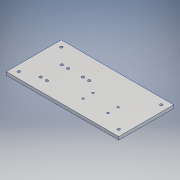
# Autodesk Inventor part: Plaque support
Saved by Autodesk Inventor 2017 (Build 210142000, 142)
## iProperties
Part Number: Plaque support
Material: Aluminium 6061
Document SubType Name: Modeling
Designer: Adrien MARY
Density: 2.7 g/cm^3
Appearance: Aluminium - Plat
Mass: 211.535 g
Surface Area: 348.794 cm^2
Volume: 78.3464 cm^3
Stock Number: 1410-02-01
Project: 1410 LaserShow
Author: Adrien MARY
Autodesk Inventor part; units mm, degrees
ref_plane "YZ Plane" through (0, 0, 0) normal (1, 0, 0) x (0, 1, 0)
ref_plane "XZ Plane" through (0, 0, 0) normal (0, 1, 0) x (-1, 0, 0)
ref_plane "XY Plane" through (0, 0, 0) normal (0, 0, 1) x (1, 0, 0)
sketch "Esquisse1" plane through (0, 0, 0) normal (0, 0, 1) x (1, 0, 0)
  line L0 (-90, -44) -> (90, -44)
  line L1 (90, -44) -> (90, 44)
  line L2 (90, 44) -> (-90, 44)
  line L3 (-90, 44) -> (-90, -44)
  line L4 (-90, -44) -> (90, 44) construction
  line L5 (90, -44) -> (-90, 44) construction
  point P0 (0, 0)
  dimension "d0" = 180
  dimension "d1" = 88
  constraints: 12 end point, 2 midpoint, 2 parallel, 1 horizontal, 1 perpendicular
  measures "d0" distance of L2.end L1.end
  measures "d1" distance of L1.end L0.end
extrude "Extrusion1" add sketch "Esquisse1" along normal mid plane 5
sketch "Esquisse2" plane through (0, 0, 2.5) normal (0, 0, 1) x (1, 0, 0)
  line L0 (-90, 44) -> (-90, -44) projected
  line L1 (90, -44) -> (-90, -44) projected
  point P0 (0, 0)
  point P1 (-45, -24)
  point P2 (-45, 9.85)
  point P3 (-11.15, 9.85)
  dimension "d4" = 33.85
  dimension "d5" = 45
  dimension "d6" = 33.85
  dimension "d7" = 20
  constraints: 1 horizontal alignment, 1 vertical alignment
  measures "d4" distance of point (-45, 9.85) point (-45, -24)
  measures "d5" distance from line of L0 point (-45, -24)
  measures "d6" distance of point (-45, 9.85) point (-11.15, 9.85)
  measures "d7" distance from line of L1 point (-45, -24)
hole "Perçage_moteur" at (-45, -24, 2.5) at (-45, 9.85, 2.5) at (-11.15, 9.85, 2.5) direction (0, 0, -1) diameter 4.2 end through all
sketch "Esquisse3" plane through (0, 0, 2.5) normal (0, 0, 1) x (1, 0, 0)
  line L0 (-60.0266, -12) -> (31.1582, -12) construction
  circle A0 centre (-45, -24) radius 2.1 construction
  circle A1 centre (-11.15, 9.85) radius 2.1 construction
  line L1 (-90, 44) -> (-90, -44) projected
  point P0 (0, 0)
  point P1 (8.85, -20)
  point P2 (8.85, -4)
  point P3 (48.85, -4)
  point P4 (48.85, -20)
  dimension "d15" = 40
  dimension "d16" = 16
  dimension "d17" = 12
  dimension "d18" = 8
  dimension "d19" = 20
  dimension "d38" = 98.85
  constraints: 2 end point, 2 horizontal alignment, 2 vertical alignment, 1 horizontal
  measures "d15" distance of point (48.85, -4) point (8.85, -4)
  measures "d16" distance of point (48.85, -20) point (48.85, -4)
  measures "d17" distance from line of L0 A0.centre
  measures "d18" distance from line of L0 point (8.85, -20)
  measures "d19" horizontal distance of A1.centre point (8.85, -4)
  measures "d38" distance from line of L1 point (8.85, -4)
hole "Perçage_laser" at (8.85, -20, 2.5) at (8.85, -4, 2.5) at (48.85, -4, 2.5) at (48.85, -20, 2.5) direction (0, 0, -1) diameter 3.2 depth 9.525 tip angle 118
sketch "Esquisse4" plane through (0, 0, 2.5) normal (0, 0, 1) x (1, 0, 0)
  line L0 (90, -44) -> (90, 44) projected
  line L1 (-90, 44) -> (90, 44) projected
  line L2 (90, -44) -> (-90, -44) projected
  line L3 (-90, 44) -> (-90, -44) projected
  point P0 (0, 0)
  point P1 (-80, -34)
  point P2 (-80, 34)
  point P3 (80, 34)
  point P4 (80, -34)
  dimension "d27" = 10
  dimension "d28" = 10
  dimension "d29" = 10
  dimension "d30" = 10
  constraints: 2 horizontal alignment, 2 vertical alignment
  measures "d27" distance from line of L0 point (80, 34)
  measures "d28" distance from line of L1 point (80, 34)
  measures "d29" distance from line of L2 point (80, -34)
  measures "d30" distance from line of L3 point (-80, -34)
hole "Perçage_coins" at (-80, -34, 2.5) at (-80, 34, 2.5) at (80, 34, 2.5) at (80, -34, 2.5) direction (0, 0, -1) diameter 4.2 depth 9.525 tip angle 118
sketch "Esquisse5" plane through (0, 0, 2.5) normal (0, 0, 1) x (1, 0, 0)
  circle A0 centre (-45, 9.85) radius 2.1 projected
  circle A1 centre (-11.15, 9.85) radius 2.1 projected
  circle A2 centre (-45, -24) radius 2.1 projected
  point P0 (0, 0)
  point P1 (-55, -24)
  point P2 (-55, 9.85)
  point P3 (-21.15, 9.85)
  dimension "d39" = 10
  dimension "d40" = 10
  dimension "d41" = 10
  constraints: 3 horizontal alignment
  measures "d39" distance of A0.centre point (-55, 9.85)
  measures "d40" distance of A1.centre point (-21.15, 9.85)
  measures "d41" distance of A2.centre point (-55, -24)
hole "Perçage4" at (-55, -24, 2.5) at (-55, 9.85, 2.5) at (-21.15, 9.85, 2.5) direction (0, 0, -1) diameter 4.2 depth 8 tip angle 118
equation "\"d18\" = 0.5 * d16"
equation "\"pi\" = 3.141593"
equation "\"nombredor\" = 1.61803"
